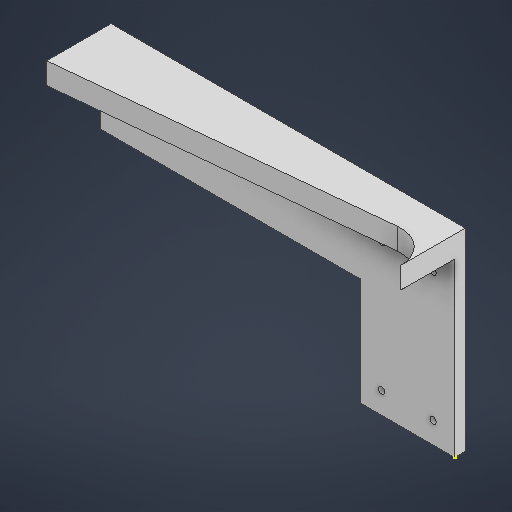
# Autodesk Inventor part: üst kısım
Saved by Autodesk Inventor 2026.1 (Build 301233020, 233B)
## iProperties
Created: 2026-04-18
Part Number: üst kısım
Material: Generic
Document SubType Name: Modeling
Designer: kadir
Density: 1 g/cm^3
Appearance: Default
Author: kadir
Autodesk Inventor part; units mm, degrees
ref_plane "YZ Plane" through (0, 0, 0) normal (1, 0, 0) x (0, 1, 0)
ref_plane "XZ Plane" through (0, 0, 0) normal (0, 1, 0) x (-1, 0, 0)
sketch "Sketch1" plane through (0, 0, 0) normal (0, 0, 1) x (1, 0, 0)
  line L0 (0, 0) -> (-44, 0)
  line L1 (-44, 0) -> (-44, 90)
  line L2 (-44, 90) -> (0, 90)
  line L3 (0, 90) -> (0, 0)
  line L4 (-44, 90) -> (-165, 90)
  line L5 (-165, 90) -> (-165, 50)
  line L6 (-165, 50) -> (-44, 50)
  line L7 (-44, 50) -> (-44, 90)
  point P0 (-44, 50)
  dimension "d0" = 44
  dimension "d1" = 90
  dimension "d2" = 40
  dimension "d3" = 121
  constraints: 16 end point, 4 parallel, 2 horizontal, 2 perpendicular
  measures "d0" distance of L1.end L2.end
  measures "d1" distance of L0.end L1.end
  measures "d2" distance of L5.end L4.end
  measures "d3" distance of L5.end L6.end
extrude "Extrusion1" add sketch "Sketch1" along normal blind 5
sketch "Sketch2" plane through (0, 0, 5) normal (0, 0, 1) x (1, 0, 0)
  point P0 (0, 0)
ref_plane "Work Plane1" through (-165, 90, 5) normal (0, 1, 0) x (1, 0, 0)
sketch "Sketch3" plane through (-165, 90, 5) normal (0, 1, 0) x (1, 0, 0)
  circle A0 centre (150, -25) radius 15
  arc A1 (7.1929, -25.7193) -> (7.1925, -24.2771) centre (0, -25) ccw
  line L0 (165, 0) -> (0.2186, 0)
  line L1 (165, 5) -> (165, -44.7143)
  line L2 (150, -40) -> (0, -25)
  line L3 (0, -25) -> (148.5, -10.0752)
  line L4 (0, 0) -> (121, 0) projected
  line L5 (165, -44.7143) -> (0, -44.7143)
  line L6 (0, -44.7143) -> (0, 0)
  line L7 (0, 0) -> (165, 0)
  line L8 (165, 0) -> (165, -44.7143)
  line L9 (0, 0) -> (0, -44.7143)
  point P0 (0, -25)
  point P1 (165, -25)
  dimension "d6" = 30
  dimension "d7" = 150
  dimension "d8" = 165
  dimension "d9" = 25
  constraints: 18 end point, 4 point on circle, 3 equal length, 3 point on line, 2 centre point, 2 horizontal, 2 tangent, 1 coincident, 1 perpendicular, 1 vertical
  measures "d6" diameter of A0
  measures "d7" distance of L2.end A0.centre
  measures "d8" distance from line of L1 L2.end
  measures "d9" distance from line of L0 A0.centre
extrude "Extrusion2" add sketch "Sketch3" against normal blind 10 contours A0 L3 L6 L4 L0 L1
sketch "Sketch4" plane through (0, 0, 5) normal (0, 0, 1) x (1, 0, 0)
  line L0 (-5, 5) -> (-15, 5)
  line L1 (-15, 5) -> (-15, 15)
  line L2 (-15, 15) -> (-5, 15)
  line L3 (-5, 15) -> (-5, 5)
  line L4 (-5, 5) -> (-15, 15) construction
  line L5 (-15, 5) -> (-5, 15) construction
  line L6 (-44, 0) -> (0, 0) projected
  line L7 (0, 0) -> (0, 80) projected
  line L8 (-22, 0) -> (-22, 96.74)
  line L9 (0, 80) -> (-165, 80) projected
  line L10 (-39, 5) -> (-29, 5)
  line L11 (-29, 5) -> (-29, 15)
  line L12 (-29, 15) -> (-39, 15)
  line L13 (-39, 15) -> (-39, 5)
  line L14 (-5, 65) -> (-15, 65)
  line L15 (-15, 65) -> (-15, 75)
  line L16 (-15, 75) -> (-5, 75)
  line L17 (-5, 75) -> (-5, 65)
  line L18 (-5, 65) -> (-15, 75) construction
  line L19 (-15, 65) -> (-5, 75) construction
  line L20 (-39, 65) -> (-29, 65)
  line L21 (-29, 65) -> (-29, 75)
  line L22 (-29, 75) -> (-39, 75)
  line L23 (-39, 75) -> (-39, 65)
  line L24 (-140, 60) -> (-150, 60)
  line L25 (-150, 60) -> (-150, 70)
  line L26 (-150, 70) -> (-140, 70)
  line L27 (-140, 70) -> (-140, 60)
  line L28 (-140, 60) -> (-150, 70) construction
  line L29 (-150, 60) -> (-140, 70) construction
  line L30 (-165, 50) -> (-44, 50) projected
  line L31 (-165, 80) -> (-165, 50) projected
  circle A0 centre (-10, 10) radius 1.5
  circle A1 centre (-10, 70) radius 1.5
  circle A2 centre (-34, 10) radius 1.5
  circle A3 centre (-34, 70) radius 1.5
  circle A4 centre (-145, 65) radius 1.5
  dimension "d12" = 10
  dimension "d13" = 10
  dimension "d14" = 10
  dimension "d15" = 10
  dimension "d16" = 10
  dimension "d17" = 10
  dimension "d18" = 10
  dimension "d19" = 10
  dimension "d20" = 10
  dimension "d21" = 15
  dimension "d22" = 20
  dimension "d23" = 3
  dimension "d24" = 3
  dimension "d25" = 3
  constraints: 54 end point, 10 symmetric about line, 7 midpoint, 6 parallel, 5 centre point, 4 perpendicular, 3 coincident, 3 horizontal, 2 other
  measures "d12" distance of L1.end L2.end
  measures "d13" distance of L0.end L1.end
  measures "d14" distance from line of L6 point (-10, 10)
  measures "d15" distance from line of L7 point (-10, 10)
  measures "d16" distance of L15.end L16.end
  measures "d17" distance of L14.end L15.end
  measures "d18" distance from line of point (-10, 70) L9
  measures "d19" distance of L25.end L26.end
  measures "d20" distance of L24.end L25.end
  measures "d21" distance from line of L30 point (-145, 65)
  measures "d22" distance from line of L31 point (-145, 65)
  measures "d23" diameter of A0
  measures "d24" diameter of A1
  measures "d25" diameter of A4
extrude "Extrusion3" cut sketch "Sketch4" against normal through all contours A0 | A1
extrude "Extrusion4" cut sketch "Sketch4" against normal through all contours A3
extrude "Extrusion5" cut sketch "Sketch4" against normal through all contours A2
extrude "Extrusion6" cut sketch "Sketch4" against normal through all contours A4
sketch "Sketch5" plane through (0, 0, 0) normal (0, 0, -1) x (-1, 0, 0)
  line L0 (5, 15) -> (15, 15)
  line L1 (15, 15) -> (15, 5)
  line L2 (15, 5) -> (5, 5)
  line L3 (5, 5) -> (5, 15)
  circle A0 centre (10, 10) radius 1.5 projected
  line L4 (5, 15) -> (15, 5) construction
  line L5 (15, 15) -> (5, 5) construction
  line L6 (5, 75) -> (15, 75)
  line L7 (15, 75) -> (15, 65)
  line L8 (15, 65) -> (5, 65)
  line L9 (5, 65) -> (5, 75)
  circle A1 centre (10, 70) radius 1.5 projected
  line L10 (5, 75) -> (15, 65) construction
  line L11 (15, 75) -> (5, 65) construction
  line L12 (44, 0) -> (0, 0) projected
  line L13 (22, 0) -> (22, 89.9769)
  line L14 (39, 15) -> (29, 15)
  line L15 (29, 15) -> (29, 5)
  line L16 (29, 5) -> (39, 5)
  line L17 (39, 5) -> (39, 15)
  circle A2 centre (34, 10) radius 1.5
  line L18 (39, 15) -> (29, 5) construction
  line L19 (29, 15) -> (39, 5) construction
  line L20 (39, 75) -> (29, 75)
  line L21 (29, 75) -> (29, 65)
  line L22 (29, 65) -> (39, 65)
  line L23 (39, 65) -> (39, 75)
  circle A3 centre (34, 70) radius 1.5
  line L24 (39, 75) -> (29, 65) construction
  line L25 (29, 75) -> (39, 65) construction
  line L26 (140, 70) -> (150, 70)
  line L27 (150, 70) -> (150, 60)
  line L28 (150, 60) -> (140, 60)
  line L29 (140, 60) -> (140, 70)
  circle A4 centre (145, 65) radius 1.5 projected
  line L30 (140, 70) -> (150, 60) construction
  line L31 (150, 70) -> (140, 60) construction
  circle A5 centre (10, 10) radius 1.5
  circle A6 centre (10, 70) radius 1.5
  circle A7 centre (34, 70) radius 1.5
  circle A8 centre (34, 10) radius 1.5
  circle A9 centre (145, 65) radius 1.5
  dimension "d34" = 10
  dimension "d35" = 10
  dimension "d36" = 10
  dimension "d37" = 10
  dimension "d38" = 10
  dimension "d39" = 10
  dimension "d40" = 3
  dimension "d41" = 3
  dimension "d42" = 3
  dimension "d43" = 3
  dimension "d44" = 3
  constraints: 62 end point, 10 symmetric about line, 7 centre point, 7 midpoint, 6 parallel, 5 coincident, 3 horizontal, 3 perpendicular, 1 vertical, 2 other
  measures "d34" distance of L1.end L2.end
  measures "d35" distance of L0.end L1.end
  measures "d36" distance of L7.end L8.end
  measures "d37" distance of L6.end L7.end
  measures "d38" distance of L27.end L28.end
  measures "d39" distance of L26.end L27.end
  measures "d40" diameter of A5
  measures "d41" diameter of A6
  measures "d42" diameter of A7
  measures "d43" diameter of A8
  measures "d44" diameter of A9
extrude "Extrusion7" cut sketch "Sketch5" against normal blind 2
body "Solid1"
